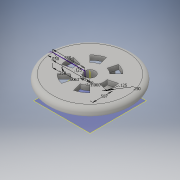
# Autodesk Inventor part: Sun_wheel
Saved by Autodesk Inventor 2016 (Build 200138000, 138)
## iProperties
Created: 2018-01-11
Part Number: Sun_wheel
Material: Generic
Document SubType Name: Modeling
Designer: sun01147
Density: 1 g/cm^3
Appearance: Default
Mass: 11.6717 g
Surface Area: 64.2946 cm^2
Volume: 11.6717 cm^3
Author: sun01147
Autodesk Inventor part; units mm, degrees
ref_plane "XZ Plane" through (0, 0, 0) normal (0, 1, 0) x (-1, 0, 0)
ref_plane "XY Plane" through (0, 0, 0) normal (0, 0, 1) x (1, 0, 0)
sketch "wheel1" plane through (0, 0, 0) normal (0, 0, 1) x (1, 0, 0)
  line L0 (-15.948, 2.7835) -> (-15.948, 2.7835)
  line L1 (-5.6765, 2.7938) -> (-5.6765, 2.7732)
  constraints: 4 end point, 2 vertical
sketch "wheel2" plane through (0, 0, 0) normal (0, 0, 1) x (1, 0, 0)
  arc A0 (-25.4, 3.175) -> (-25.4, -3.175) centre (-25.4, 0) ccw
  line L0 (-25.4, 3.175) -> (-3.556, 3.175)
  line L1 (-3.556, 3.175) -> (-3.556, -3.175)
  line L2 (-25.4, -3.175) -> (-25.4, 3.175) construction
  line L3 (-19.05, -3.175) -> (-6.35, -3.175) construction
  line L4 (-6.35, -1.5875) -> (-6.35, -1.5875)
  line L5 (-7.9375, 0) -> (-17.4625, 0)
  line L6 (-19.05, -1.5875) -> (-19.05, -1.5875)
  line L7 (-3.556, -3.175) -> (-4.7625, -3.175)
  line L8 (-20.6375, -3.175) -> (-25.4, -3.175)
  arc A1 (-20.6375, -3.175) -> (-19.05, -1.5875) centre (-20.6375, -1.5875) ccw
  arc A2 (-6.35, -1.5875) -> (-4.7625, -3.175) centre (-4.7625, -1.5875) ccw
  arc A3 (-17.4625, 0) -> (-19.05, -1.5875) centre (-17.4625, -1.5875) ccw
  arc A4 (-6.35, -1.5875) -> (-7.9375, 0) centre (-7.9375, -1.5875) ccw
  line L9 (0, -4.8395) -> (0, 4.5108) projected
  point P0 (0, 0)
  point P1 (-6.35, 0)
  dimension "d35" = 6.35
  dimension "d36" = 25.4
  dimension "d37" = 21.844
  dimension "d39" = 3.175
  dimension "d40" = 6.35
  dimension "d41" = 6.35
  dimension "d42" = 3.175
  dimension "d43" = 1.5875
  constraints: 18 end point, 10 point on circle, 8 tangent, 6 point on line, 5 centre point, 5 parallel, 3 equal radius, 2 horizontal, 2 perpendicular, 1 horizontal alignment
  measures "d35" diameter of A0
  measures "d36" distance of point (0, 0) A0.centre
  measures "d37" distance of L0.start L0.end
  measures "d39" distance of point (-6.35, 0) L3.end
  measures "d40" distance between parallel lines of L2 L6
  measures "d41" distance from line of point (0, 0) L4
  measures "d42" distance between parallel lines of L5 L0
  measures "d43" radius of A1
revolve "Revolution1" add sketch "wheel2" angle 360 about axis through (0, -10, 0) along (0, 1, 0)
sketch "Sketch6" plane through (0, 0, 0) normal (0, -1, 0) x (1, 0, 0)
  circle A0 centre (0, 0) radius 7.9375 projected
  circle A1 centre (0, 0) radius 17.4625 projected
  arc A2 (15.3341, -4.1088) -> (15.3341, 4.1088) centre (0, 0) ccw
  arc A3 (9.2004, -2.4653) -> (9.2004, 2.4653) centre (0, 0) ccw
  line L0 (9.2004, 2.4653) -> (15.3341, 4.1088)
  line L1 (9.2004, -2.4653) -> (15.3341, -4.1088)
  arc A4 (11.2253, 11.2253) -> (4.1088, 15.3341) centre (0, 0) ccw
  line L2 (2.4653, 9.2004) -> (4.1088, 15.3341)
  arc A5 (6.7352, 6.7352) -> (2.4653, 9.2004) centre (0, 0) ccw
  line L3 (6.7352, 6.7352) -> (11.2253, 11.2253)
  arc A6 (-4.1088, 15.3341) -> (-11.2253, 11.2253) centre (0, 0) ccw
  line L4 (-6.7352, 6.7352) -> (-11.2253, 11.2253)
  arc A7 (-2.4653, 9.2004) -> (-6.7352, 6.7352) centre (0, 0) ccw
  line L5 (-2.4653, 9.2004) -> (-4.1088, 15.3341)
  arc A8 (-15.3341, 4.1088) -> (-15.3341, -4.1088) centre (0, 0) ccw
  line L6 (-9.2004, -2.4653) -> (-15.3341, -4.1088)
  arc A9 (-9.2004, 2.4653) -> (-9.2004, -2.4653) centre (0, 0) ccw
  line L7 (-9.2004, 2.4653) -> (-15.3341, 4.1088)
  arc A10 (-11.2253, -11.2253) -> (-4.1088, -15.3341) centre (0, 0) ccw
  line L8 (-2.4653, -9.2004) -> (-4.1088, -15.3341)
  arc A11 (-6.7352, -6.7352) -> (-2.4653, -9.2004) centre (0, 0) ccw
  line L9 (-6.7352, -6.7352) -> (-11.2253, -11.2253)
  arc A12 (4.1088, -15.3341) -> (11.2253, -11.2253) centre (0, 0) ccw
  line L10 (6.7352, -6.7352) -> (11.2253, -11.2253)
  arc A13 (2.4653, -9.2004) -> (6.7352, -6.7352) centre (0, 0) ccw
  line L11 (2.4653, -9.2004) -> (4.1088, -15.3341)
  dimension "d47" = 31.75
  dimension "d48" = 19.05
  dimension "d51" = 360
  constraints: 24 end point, 24 point on circle, 12 centre point, 7 coincident, 61 other
  measures "d47" diameter of A2
  measures "d48" diameter of A3
extrude "Extrusion2" cut sketch "Sketch6" against normal blind 6.35 contours L1 A3 L0 A2 | L3 A5 L2 A4 | L5 A7 L4 A6 | L7 A9 L6 A8 | L9 A11 L8 A10 | L11 A13 L10 A12
ref_plane "Work Plane1" through (0, -12.7, 0) normal (0, -1, 0) x (1, 0, 0)
sketch "wheel3" plane through (0, -3.175, 0) normal (0, -1, 0) x (1, 0, 0)
  point P0 (0, 0)
sketch "wheel5" plane through (0, -12.7, 0) normal (0, -1, 0) x (1, 0, 0)
  circle A0 centre (0, -12.8814) radius 3.175
  circle A1 centre (0, -12.8814) radius 1.5875
  point P0 (0, 0)
  dimension "d58" = 6.35
  dimension "d61" = 3.175
  dimension "d67" = 12.8814
  constraints: 2 centre point, 1 coincident, 1 vertical alignment
  measures "d58" diameter of A0
  measures "d61" diameter of A1
  measures "d67" distance of A0.centre point (0, 0)
extrude "Extrusion3" add sketch "wheel5" against normal up to next contours A0 | A1
extrude "Extrusion4" add sketch "wheel5" along normal blind 3.175 contours A1
sketch "Sketch12" plane through (0, -12.7, 0) normal (0, -1, 0) x (1, 0, 0)
  point P0 (0, 0)
sketch "Sketch13" plane through (0, -15.875, -12.8814) normal (0, -1, 0) x (1, 0, 0)
  circle A0 centre (0, 0) radius 1.5875 projected
  point P0 (0, 12.8814)
hole "Hole1" at (0, -15.875, -12.8814) direction (0, 1, 0) diameter 1.5875 depth 6.35 tip angle 118
body "Solid2"
